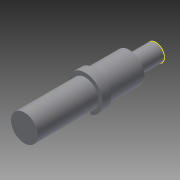
# Autodesk Inventor part: driving_shaft
Saved by Autodesk Inventor 2016 (Build 200138000, 138)
## iProperties
Created: 2015-09-10
Part Number: driving_shaft
Material: Generic
Document SubType Name: Modeling
Designer: Students
Density: 1 g/cm^3
Appearance: Default
Author: Students
Autodesk Inventor part; units mm, degrees
ref_plane "YZ Plane" through (0, 0, 0) normal (1, 0, 0) x (0, 1, 0)
ref_plane "XZ Plane" through (0, 0, 0) normal (0, 1, 0) x (-1, 0, 0)
ref_plane "XY Plane" through (0, 0, 0) normal (0, 0, 1) x (1, 0, 0)
sketch "Sketch1" plane through (0, 0, 0) normal (0, 1, 0) x (-1, 0, 0)
  point P0 (0, 0)
sketch "Sketch2" plane through (0, 0, 0) normal (0, 1, 0) x (-1, 0, 0)
  circle A0 centre (0, 0) radius 10
  dimension "d0" = 20
  constraints: 1 centre point, 1 coincident
  measures "d0" diameter of A0
extrude "Extrusion1" add sketch "Sketch2" along normal blind 5
sketch "Sketch3" plane through (0, 5, 0) normal (0, 1, 0) x (1, 0, 0)
  circle A0 centre (0, 0) radius 10 projected
  circle A1 centre (0, 0) radius 8.6
  dimension "d3" = 17.2
  constraints: 1 centre point, 1 coincident
  measures "d3" diameter of A1
extrude "Extrusion2" add sketch "Sketch3" along normal blind 20.5 contours A1
sketch "Sketch4" plane through (0, 25.5, 0) normal (0, 1, 0) x (1, 0, 0)
  circle A0 centre (0, 0) radius 8.6 projected
  circle A1 centre (0, 0) radius 5
  dimension "d6" = 10
  constraints: 1 centre point, 1 coincident
  measures "d6" diameter of A1
extrude "Extrusion3" add sketch "Sketch4" along normal blind 15 contours A1
sketch "Sketch5" plane through (0, 0, 0) normal (0, -1, 0) x (1, 0, 0)
  circle A0 centre (0, 0) radius 10 projected
  circle A1 centre (0, 0) radius 7.7
  dimension "d9" = 15.4
  constraints: 1 centre point, 1 coincident
  measures "d9" diameter of A1
extrude "Extrusion4" add sketch "Sketch5" along normal blind 35 contours A1
sketch "Sketch6" plane through (0, 25.5, 0) normal (0, 1, 0) x (1, 0, 0)
  line L0 (0, 9.9966) -> (0, 6.4466)
  line L1 (0, 6.4466) -> (3, 6.4466)
  line L2 (3, 6.4466) -> (-3, 6.4466)
  line L3 (-3, 6.4466) -> (-3, 9.9966)
  line L4 (-3, 9.9966) -> (3, 9.9966)
  line L5 (3, 9.9966) -> (3, 6.4466)
  dimension "d13" = 3.55
  dimension "d14" = 3
  dimension "d15" = 6
  dimension "d16" = 3.55
  constraints: 12 end point, 2 parallel, 2 perpendicular, 1 horizontal, 1 vertical
  measures "d13" distance of L0.start L0.end
  measures "d14" distance of L0.end L1.end
  measures "d15" distance of L3.end L4.end
  measures "d16" distance of L2.end L3.end
sketch "Sketch7" plane through (0, 40.5, 0) normal (0, 1, 0) x (1, 0, 0)
  circle A0 centre (0, 0) radius 5 projected
extrude "Extrusion5" cut sketch "Sketch6" against normal blind 25.5
body "Solid1"
